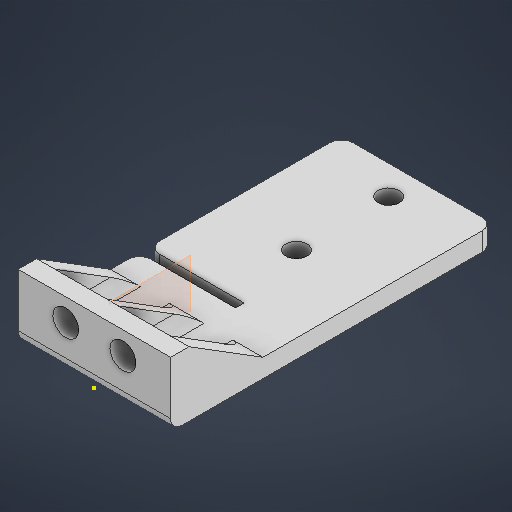
# Autodesk Inventor part: для захвата
Saved by Autodesk Inventor 2025 (Build 290162000, 162)
## iProperties
Created: 2025-02-15
Part Number: для захвата
Material: Типовые
Document SubType Name: Modeling
Designer: Phantom
Density: 1 g/cm^3
Appearance: По умолчанию
Author: Phantom
Autodesk Inventor part; units mm, degrees
ref_plane "YZ Plane" through (0, 0, 0) normal (1, 0, 0) x (0, 1, 0)
ref_plane "XZ Plane" through (0, 0, 0) normal (0, 1, 0) x (-1, 0, 0)
ref_plane "XY Plane" through (0, 0, 0) normal (0, 0, 1) x (1, 0, 0)
sketch "Эскиз1" plane through (0, 0, 0) normal (0, 1, 0) x (-1, 0, 0)
  circle A0 centre (0, 8) radius 1.85
  circle A1 centre (0, -8) radius 1.85
  line L0 (0, -8) -> (0, -13)
  line L1 (0, -13) -> (5, -13)
  line L2 (5, -13) -> (5, 43)
  line L3 (5, 43) -> (0, 43)
  line L4 (0, 43) -> (0, -13)
  line L5 (0, -13) -> (-5, -13)
  line L6 (-5, -13) -> (-5, 43)
  line L7 (-5, 43) -> (0, 43)
  line L8 (5, -13) -> (10, -13)
  line L9 (10, -13) -> (10, 43)
  line L10 (10, 43) -> (5, 43)
  line L11 (5, 43) -> (5, -13)
  line L12 (-5, -13) -> (-10, -13)
  line L13 (-10, -13) -> (-10, 43)
  line L14 (-10, 43) -> (-5, 43)
  line L15 (-5, 43) -> (-5, -13)
  point P0 (0, 0)
  dimension "d0" = 5
  dimension "d2" = 56
  constraints: 32 end point, 6 parallel, 3 horizontal, 3 perpendicular, 2 centre point, 2 symmetric about line, 1 point on line, 1 vertical
  measures "d0" distance of L0.start L0.end
  measures "d2" distance of L1.end L2.end
extrude "Выдавливание1" add sketch "Эскиз1" along normal blind 3.2 contours A0 L4 L3 L2 L1 L0 A1 | A0 L4 A1 L0 L5 L6 L7 | L10 L9 L8 L2 | L6 L12 L13 L14
sketch "Эскиз2" plane through (0, 0, 0) normal (0, -1, 0) x (1, 0, 0)
  line L0 (-10, 43) -> (10, 43) projected
  line L1 (-10, 43) -> (10, 43)
  line L2 (10, 43) -> (10, 39.8)
  line L3 (10, 39.8) -> (-10, 39.8)
  line L4 (-10, 39.8) -> (-10, 43)
  point P0 (0, 0)
  dimension "d9" = 20
  dimension "d10" = 3.2
  constraints: 8 end point, 2 parallel, 1 horizontal, 1 perpendicular
  measures "d9" distance of L2.end L3.end
  measures "d10" distance of L1.end L2.end
extrude "Выдавливание2" add sketch "Эскиз2" against normal blind 10
sketch "Эскиз3" plane through (0, 10, 0) normal (0, 1, 0) x (1, 0, 0)
  line L0 (10, -39.8) -> (-10, -39.8) projected
  line L1 (-10, -39.8) -> (-10, -43) projected
  line L2 (-10, -43) -> (10, -43) projected
  line L3 (10, -43) -> (10, -39.8) projected
  point P0 (0, 0)
extrude "Выдавливание3" add sketch "Эскиз3" along normal blind 1.2
sketch "Эскиз4" plane through (-10, 0, 43) normal (0, 0, 1) x (1, 0, 0)
  point P0 (10, 0)
sketch "Эскиз5" plane through (-10, 0, 43) normal (0, 0, 1) x (1, 0, 0)
  ellipse E0 centre (5.0518, 7.3165) end of major axis (5.0518, 5.0665) minor radius 2.25 (7.0518, 6.2858) -> (3.0519, 6.2858) ccw projected
  ellipse E1 centre (14.9518, 7.3165) end of major axis (14.9518, 9.5665) minor radius 2.25 (16.9518, 6.2858) -> (12.9518, 6.2858) ccw projected
  circle A0 centre (5.0518, 7.3165) radius 2.25
  circle A1 centre (14.9518, 7.3165) radius 2.25
  point P0 (10, 0)
  point P1 (14.9518, 9.5665)
  point P2 (16.9518, 6.2858)
  point P3 (5.031, 9.5664)
  point P4 (5.0518, 9.5665)
  constraints: 2 centre point, 2 coincident, 4 other
extrude "Выдавливание4" cut sketch "Эскиз5" against normal through all
sketch "Эскиз6" plane through (10, 0, 43) normal (1, 0, 0) x (0, 0, -1)
  line L0 (0, 0) -> (56, 0) projected
  line L1 (56, 0) -> (56, 3.2) projected
  line L2 (3.2, 3.2) -> (56, 3.2) projected
  line L3 (3.2, 3.2) -> (3.2, 11.2) projected
  line L4 (0, 11.2) -> (3.2, 11.2) projected
  line L5 (0, 0) -> (0, 11.2) projected
  line L6 (3.2, 11.2) -> (16, 3.2)
  point P0 (43, 0)
  constraints: 2 end point, 1 point on line
extrude "Выдавливание5" add sketch "Эскиз6" along normal blind 3.2
sketch "Эскиз7" plane through (-10, 0, -13) normal (-1, 0, 0) x (0, 0, 1)
  line L0 (52.8, 3.2) -> (52.8, 11.2) projected
  line L1 (40, 3.2) -> (52.8, 11.2) projected
  line L2 (52.8, 3.2) -> (40, 3.2) projected
  line L3 (0, 3.2) -> (52.8, 3.2) projected
  line L4 (0, 0) -> (0, 3.2) projected
  line L5 (0, 0) -> (56, 0) projected
  line L6 (56, 0) -> (56, 11.2) projected
  line L7 (52.8, 11.2) -> (56, 11.2) projected
  line L8 (52.8, 3.2) -> (52.8, 11.2) projected
  point P0 (13, 0)
extrude "Выдавливание6" add sketch "Эскиз7" along normal blind 3.2
ref_plane "РабПлоскость1" through (0, 0, -13) normal (1, 0, 0) x (0, 0, -1)
sketch "Эскиз8" plane through (0, 0, -13) normal (1, 0, 0) x (0, 0, -1)
  line L0 (-40, 3.2) -> (-52.8, 3.2) projected
  line L1 (-52.8, 11.2) -> (-40, 3.2) projected
  line L2 (-52.8, 3.2) -> (-52.8, 11.2) projected
  point P0 (-13, 0)
extrude "Выдавливание7" add sketch "Эскиз8" along normal blind 1
sketch "Эскиз9" plane through (0, 0, -13) normal (-1, 0, 0) x (0, 0, 1)
  line L0 (52.8, 11.2) -> (52.8, 3.2) projected
  line L1 (40, 3.2) -> (52.8, 11.2) projected
  line L2 (52.8, 3.2) -> (40, 3.2) projected
  point P0 (13, 0)
extrude "Выдавливание8" add sketch "Эскиз9" along normal blind 1
fillet "Сопряжение1" radius 2 4 edges at (10, 3.2, 33.4) (-10, 3.2, 33.4) (1, 3.2, 33.4) (-1, 3.2, 33.4)
sketch "Эскиз10" plane through (0, 0, 0) normal (0, -1, 0) x (1, 0, 0)
  line L0 (-3.5723, 19.4902) -> (-3.5624, 22.9902) projected
  arc A0 (3.4361, 23.0104) -> (2.939, 23.4718) centre (2.9376, 22.9718) ccw projected
  line L1 (8.9377, 22.9949) -> (3.4361, 23.0104) projected
  line L2 (8.9941, 42.9548) -> (8.9377, 22.9949) projected
  line L3 (-9.0058, 43.0057) -> (8.9941, 42.9548) projected
  line L4 (-9.0058, 43.0057) -> (-9.0623, 23.0457) projected
  line L5 (-3.5607, 23.0302) -> (-9.0623, 23.0457) projected
  arc A1 (-3.061, 23.4888) -> (-3.5607, 23.0302) centre (-3.0624, 22.9888) ccw projected
  line L6 (-3.061, 23.4888) -> (2.939, 23.4718) projected
  line L7 (-3.5723, 19.4902) -> (-3.5624, 22.9902) projected
  line L8 (-9.0624, 23.0057) -> (-3.5624, 22.9902) projected
  line L9 (-9.0736, 19.0258) -> (-9.0624, 23.0057) projected
  line L10 (-3.2137, 19.0092) -> (-9.0736, 19.0258) projected
  arc A2 (-3.5723, 19.4902) -> (-3.2137, 19.0092) centre (-3.0723, 19.4888) ccw projected
  arc A3 (3.0663, 18.9914) -> (3.4277, 19.4704) centre (2.9277, 19.4718) ccw projected
  line L11 (8.9263, 18.9749) -> (3.0663, 18.9914) projected
  line L12 (8.9263, 18.9749) -> (8.9376, 22.9549) projected
  line L13 (3.4376, 22.9704) -> (8.9376, 22.9549) projected
  line L14 (3.4376, 22.9704) -> (3.4277, 19.4704) projected
  line L15 (-8.4673, 17.424) -> (-5.3782, 17.4153) projected
  line L16 (-5.3782, 17.4153) -> (-5.3821, 16.0153) projected
  line L17 (-5.3821, 16.0153) -> (5.2178, 15.9853) projected
  line L18 (5.2178, 15.9853) -> (5.2218, 17.3853) projected
  line L19 (5.2218, 17.3853) -> (8.3109, 17.3766) projected
  line L20 (9.0056, 18.9674) -> (8.3109, 17.3766) projected
  ellipse E0 centre (8.9198, 16.6672) end of major axis (8.9263, 18.9749) minor radius 1 (9.0056, 18.9674) -> (8.9263, 18.9749) ccw projected
  line L21 (8.9263, 18.9749) -> (3.0663, 18.9914) projected
  line L22 (3.0663, 18.9914) -> (-3.2137, 19.0092) projected
  line L23 (-3.2137, 19.0092) -> (-9.0736, 19.0258) projected
  ellipse E1 centre (-9.0802, 16.7181) end of major axis (-9.0736, 19.0258) minor radius 1 (-9.0736, 19.0258) -> (-9.1529, 19.0187) ccw projected
  line L24 (-8.4673, 17.424) -> (-9.1529, 19.0187) projected
  line L25 (3.4376, 23.4704) -> (-15, 23.4704)
  line L26 (-15, 23.4704) -> (-15, 18.9749)
  line L27 (-15, 18.9749) -> (3.4376, 18.9749)
  line L28 (3.4376, 18.9749) -> (3.4376, 23.4704)
  point P0 (0, 0)
  constraints: 8 end point, 2 parallel, 1 horizontal, 1 perpendicular, 2 other
extrude "Выдавливание9" cut sketch "Эскиз10" against normal through all contours A2 L10 L9 L8 L0 | L0 L8 L9 E1 L24 L27 L26 L25 L4 L5 A1 A0 L28 L14 A3 L22 A2 | L22 L11 L28 L27 L24 E1 L10 | A3 L14 L28 L11 | A0 L25 L28 | L25 A1 L5 L4
fillet "Сопряжение2" radius 2 2 edges at (3.4376, 1.6, 23.4704) (3.4376, 1.6, 18.9749)
fillet "Сопряжение3" radius 2 4 edges at (13.2, 1.6, -13) (-13.2, 1.6, -13) (-13.2, 1.6, 23.4704) (-13.2, 1.6, 18.9749)
fillet "Сопряжение4" radius 2 1 edges at (0, 0, 43)
sketch "Эскиз11" plane through (0, 0, 0) normal (0, -1, 0) x (1, 0, 0)
  line L0 (3.4376, 21.4704) -> (3.4376, 20.9749) projected
  line L1 (3.4376, 21.2226) -> (-14.4424, 21.2226)
  line L2 (3.4376, 21.2226) -> (-13.5624, 21.2226)
  line L3 (-13.5624, 21.2226) -> (-13.5624, 21.9726)
  line L4 (-13.5624, 21.9726) -> (3.4376, 21.9726)
  line L5 (3.4376, 21.9726) -> (3.4376, 21.2226)
  line L6 (-13.5624, 21.2226) -> (-13.5624, 20.4726)
  line L7 (-13.5624, 20.4726) -> (3.4376, 20.4726)
  line L8 (3.4376, 20.4726) -> (3.4376, 21.2226)
  circle A0 centre (0, -8) radius 1.85 projected
  circle A1 centre (0, 8) radius 1.85 projected
  line L9 (-13.2, 41) -> (13.2, 41) projected
  line L10 (-13.2, 25.4704) -> (-13.2, 41) projected
  arc A2 (-13.2, 25.4704) -> (-11.2, 23.4704) centre (-11.2, 25.4704) ccw projected
  line L11 (-11.2, 23.4704) -> (1.4376, 23.4704) projected
  arc A3 (3.4376, 21.4704) -> (1.4376, 23.4704) centre (1.4376, 21.4704) ccw projected
  line L12 (3.4376, 21.4704) -> (3.4376, 20.9749) projected
  arc A4 (1.4376, 18.9749) -> (3.4376, 20.9749) centre (1.4376, 20.9749) ccw projected
  line L13 (1.4376, 18.9749) -> (-11.2, 18.9749) projected
  arc A5 (-11.2, 18.9749) -> (-13.2, 16.9749) centre (-11.2, 16.9749) ccw projected
  line L14 (-13.2, -11) -> (-13.2, 16.9749) projected
  arc A6 (-13.2, -11) -> (-11.2, -13) centre (-11.2, -11) ccw projected
  line L15 (-11.2, -13) -> (11.2, -13) projected
  arc A7 (11.2, -13) -> (13.2, -11) centre (11.2, -11) ccw projected
  line L16 (13.2, 41) -> (13.2, -11) projected
  line L17 (-13.2, 16.9749) -> (-13.2, -11) projected
  line L18 (-13.2, 25.4704) -> (-13.2, 16.9749)
  point P0 (0, 0)
  point P1 (-13.2, 21.9726)
  point P2 (3.3735, 21.9726)
  point P3 (3.3735, 20.4726)
  point P4 (-13.2, 20.4726)
  dimension "d30" = 17
  dimension "d31" = 0.75
  constraints: 18 end point, 2 horizontal, 2 parallel, 2 symmetric about line, 1 midpoint, 1 perpendicular, 1 vertical
  measures "d30" distance of L3.end L4.end
  measures "d31" distance of L2.end L3.end
extrude "Выдавливание10" add sketch "Эскиз11" against normal up to surface (3.2 mm away) contours L4 L18 A2 L11 A3 | A4 L13 A5 L18 L7
fillet "Сопряжение5" radius 2 2 edges at (-13.2, 1.6, 20.4726) (-13.2, 1.6, 21.9726)
